Autodesk Fusion 360 part; units mm, degrees
note: some values were not read from the file. Set by a fixed rule: which sketch regions a step uses.
(part 17 of 20)
  spline S37 degree 5 poles (12.6699, 9.771) (12.6679, 9.7705) (12.6637, 9.7696) (12.6575, 9.7682) (12.6492, 9.7663) (12.6389, 9.7639) (12.6286, 9.7615) (12.6184, 9.7591) (12.6081, 9.7566) (12.5979, 9.7542) (12.5878, 9.7518) (12.5776, 9.7493) (12.5675, 9.7469) (12.5574, 9.7444) (12.5474, 9.7419) (12.5374, 9.7394) (12.5274, 9.7369) (12.5174, 9.7344) (12.5075, 9.7319) (12.4976, 9.7293) (12.4877, 9.7268) (12.4779, 9.7243) (12.4681, 9.7217) (12.4583, 9.7191) (12.4486, 9.7166) (12.4389, 9.714) (12.4292, 9.7114) (12.4195, 9.7088) (12.4099, 9.7062) (12.4003, 9.7036) (12.3908, 9.7009) (12.3812, 9.6983) (12.3717, 9.6957) (12.3623, 9.693) (12.3528, 9.6904) (12.3434, 9.6877) (12.3341, 9.685) (12.3247, 9.6823) (12.3154, 9.6797) (12.3062, 9.677) (12.2969, 9.6743) (12.2877, 9.6716) (12.2785, 9.6688) (12.2694, 9.6661) (12.2603, 9.6634) (12.2512, 9.6607) (12.2421, 9.6579) (12.2331, 9.6552) (12.2241, 9.6524) (12.2152, 9.6496) (12.2063, 9.6469) (12.1974, 9.6441) (12.1885, 9.6413) (12.1797, 9.6385) (12.1709, 9.6357) (12.1622, 9.6329) (12.1535, 9.6301) (12.1448, 9.6273) (12.1361, 9.6245) (12.1275, 9.6217) (12.1189, 9.6189) (12.1104, 9.616) (12.1018, 9.6132) (12.0934, 9.6104) (12.0849, 9.6075) (12.0765, 9.6047) (12.0681, 9.6018) (12.0598, 9.599) (12.0515, 9.5961) (12.0432, 9.5933) (12.035, 9.5904) (12.0267, 9.5875) (12.0186, 9.5846) (12.0104, 9.5818) (12.0023, 9.5789) (11.9943, 9.576) (11.9862, 9.5731) (11.9782, 9.5702) (11.9703, 9.5673) (11.9624, 9.5644) (11.9545, 9.5615) (11.9466, 9.5586) (11.9388, 9.5557) (11.931, 9.5528) (11.9233, 9.5499) (11.9156, 9.547) (11.9079, 9.5441) (11.9002, 9.5412) (11.8926, 9.5383) (11.8851, 9.5354) (11.8776, 9.5325) (11.8701, 9.5295) (11.8626, 9.5266) (11.8552, 9.5237) (11.8478, 9.5208) (11.8405, 9.5179) (11.8332, 9.515) (11.8259, 9.512) (11.8187, 9.5091) (11.8115, 9.5062) (11.8043, 9.5033) (11.7972, 9.5004) (11.7901, 9.4975) (11.7831, 9.4945) (11.7761, 9.4916) (11.7691, 9.4887) (11.7622, 9.4858) (11.7553, 9.4829) (11.7484, 9.48) (11.7416, 9.4771) (11.7348, 9.4742) (11.7281, 9.4713) (11.7214, 9.4684) (11.7148, 9.4655) (11.7081, 9.4626) (11.7016, 9.4597) (11.695, 9.4568) (11.6885, 9.4539) (11.6821, 9.451) (11.6756, 9.4482) (11.6693, 9.4453) (11.6629, 9.4424) (11.6566, 9.4396) (11.6504, 9.4367) (11.6441, 9.4338) (11.638, 9.431) (11.6318, 9.4281) (11.6257, 9.4253) (11.6197, 9.4225) (11.6137, 9.4196) (11.6077, 9.4168) (11.6017, 9.414) (11.5959, 9.4112) (11.59, 9.4084) (11.5842, 9.4056) (11.5784, 9.4028) (11.5727, 9.4) (11.567, 9.3972) (11.5614, 9.3944) (11.5558, 9.3917) (11.5502, 9.3889) (11.5447, 9.3862) (11.5392, 9.3834) (11.5338, 9.3807) (11.5284, 9.378) (11.5231, 9.3753) (11.5178, 9.3725) (11.5125, 9.3699) (11.5073, 9.3672) (11.5021, 9.3645) (11.497, 9.3618) (11.4919, 9.3592) (11.4869, 9.3565) (11.4819, 9.3539) (11.4769, 9.3513) (11.472, 9.3487) (11.4672, 9.3461) (11.4623, 9.3435) (11.4576, 9.3409) (11.4528, 9.3383) (11.4482, 9.3358) (11.4435, 9.3332) (11.4389, 9.3307) (11.4344, 9.3282) (11.4299, 9.3257) (11.4254, 9.3232) (11.421, 9.3207) (11.4167, 9.3183) (11.4123, 9.3158) (11.4081, 9.3134) (11.4038, 9.311) (11.3997, 9.3086) (11.3955, 9.3062) (11.3915, 9.3039) (11.3874, 9.3015) (11.3834, 9.2992) (11.3795, 9.2969) (11.3756, 9.2946) (11.3718, 9.2923) (11.368, 9.2901) (11.3642, 9.2878) (11.3605, 9.2856) (11.3569, 9.2834) (11.3533, 9.2812) (11.3497, 9.2791) (11.3462, 9.2769) (11.3428, 9.2748) (11.3394, 9.2727) (11.336, 9.2706) (11.3327, 9.2685) (11.3295, 9.2665) (11.3263, 9.2645) (11.3231, 9.2625) (11.32, 9.2605) (11.317, 9.2586) (11.314, 9.2567) (11.311, 9.2548) (11.3081, 9.2529) (11.3053, 9.2511) (11.3025, 9.2492) (11.2998, 9.2474) (11.2971, 9.2457) (11.2944, 9.2439) (11.2919, 9.2422) (11.2893, 9.2405) (11.2869, 9.2389) (11.2844, 9.2372) (11.2821, 9.2356) (11.2798, 9.2341) (11.2775, 9.2325) (11.2753, 9.231) (11.2732, 9.2295) (11.2711, 9.2281) (11.269, 9.2266) (11.2671, 9.2253) (11.2651, 9.2239) (11.2633, 9.2226) (11.2615, 9.2213) (11.2597, 9.22) (11.258, 9.2188) (11.2564, 9.2177) (11.2548, 9.2165) (11.2533, 9.2154) (11.2518, 9.2143) (11.2504, 9.2133) (11.2491, 9.2123) (11.2478, 9.2113) (11.2465, 9.2104) (11.2454, 9.2096) (11.2443, 9.2087) (11.2432, 9.2079) (11.2422, 9.2072) (11.2413, 9.2065) (11.2404, 9.2058) (11.2396, 9.2052) (11.2389, 9.2046) (11.2382, 9.2041) (11.2376, 9.2036) (11.2371, 9.2032) (11.2366, 9.2028) (11.2362, 9.2025) (11.2359, 9.2022) (11.2357, 9.2021) (11.2356, 9.202) (11.2355, 9.202) knots -1 -1 -1 -1 -1 -1 -0.99583333 -0.99166667 -0.9875 -0.98333333 -0.97916667 -0.975 -0.97083333 -0.96666667 -0.9625 -0.95833333 -0.95416667 -0.95 -0.94583333 -0.94166667 -0.9375 -0.93333333 -0.92916667 -0.925 -0.92083333 -0.91666667 -0.9125 -0.90833333 -0.90416667 -0.9 -0.89583333 -0.89166667 -0.8875 -0.88333333 -0.87916667 -0.875 -0.87083333 -0.86666667 -0.8625 -0.85833333 -0.85416667 -0.85 -0.84583333 -0.84166667 -0.8375 -0.83333333 -0.82916667 -0.825 -0.82083333 -0.81666667 -0.8125 -0.80833333 -0.80416667 -0.8 -0.79583333 -0.79166667 -0.7875 -0.78333333 -0.77916667 -0.775 -0.77083333 -0.76666667 -0.7625 -0.75833333 -0.75416667 -0.75 -0.74583333 -0.74166667 -0.7375 -0.73333333 -0.72916667 -0.725 -0.72083333 -0.71666667 -0.7125 -0.70833333 -0.70416667 -0.7 -0.69583333 -0.69166667 -0.6875 -0.68333333 -0.67916667 -0.675 -0.67083333 -0.66666667 -0.6625 -0.65833333 -0.65416667 -0.65 -0.64583333 -0.64166667 -0.6375 -0.63333333 -0.62916667 -0.625 -0.62083333 -0.61666667 -0.6125 -0.60833333 -0.60416667 -0.6 -0.59583333 -0.59166667 -0.5875 -0.58333333 -0.57916667 -0.575 -0.57083333 -0.56666667 -0.5625 -0.55833333 -0.55416667 -0.55 -0.54583333 -0.54166667 -0.5375 -0.53333333 -0.52916667 -0.525 -0.52083333 -0.51666667 -0.5125 -0.50833333 -0.50416667 -0.5 -0.49583333 -0.49166667 -0.4875 -0.48333333 -0.47916667 -0.475 -0.47083333 -0.46666667 -0.4625 -0.45833333 -0.45416667 -0.45 -0.44583333 -0.44166667 -0.4375 -0.43333333 -0.42916667 -0.425 -0.42083333 -0.41666667 -0.4125 -0.40833333 -0.40416667 -0.4 -0.39583333 -0.39166667 -0.3875 -0.38333333 -0.37916667 -0.375 -0.37083333 -0.36666667 -0.3625 -0.35833333 -0.35416667 -0.35 -0.34583333 -0.34166667 -0.3375 -0.33333333 -0.32916667 -0.325 -0.32083333 -0.31666667 -0.3125 -0.30833333 -0.30416667 -0.3 -0.29583333 -0.29166667 -0.2875 -0.28333333 -0.27916667 -0.275 -0.27083333 -0.26666667 -0.2625 -0.25833333 -0.25416667 -0.25 -0.24583333 -0.24166667 -0.2375 -0.23333333 -0.22916667 -0.225 -0.22083333 -0.21666667 -0.2125 -0.20833333 -0.20416667 -0.2 -0.19583333 -0.19166667 -0.1875 -0.18333333 -0.17916667 -0.175 -0.17083333 -0.16666667 -0.1625 -0.15833333 -0.15416667 -0.15 -0.14583333 -0.14166667 -0.1375 -0.13333333 -0.12916667 -0.125 -0.12083333 -0.11666667 -0.1125 -0.10833333 -0.10416667 -0.1 -0.09583333 -0.09166667 -0.0875 -0.08333333 -0.07916667 -0.075 -0.07083333 -0.06666667 -0.0625 -0.05833333 -0.05416667 -0.05 -0.04583333 -0.04166667 -0.0375 -0.03333333 -0.02916667 -0.025 -0.02083333 -0.01666667 -0.0125 -0.00833333 -0.00416667 0 0 0 0 0 0
  line L74 (11.2355, 9.202) -> (11.235, 9.2016)
  line L75 (11.235, 9.2016) -> (10.6376, 8.7123)
  arc A46 (10.6376, 8.7123) -> (9.7765, 9.6687) centre (0, 0) ccw
  line L76 (9.7765, 9.6687) -> (10.3255, 10.2117)
  line L77 (10.3255, 10.2117) -> (10.326, 10.2121)
  spline S38 degree 5 poles (10.326, 10.2121) (10.326, 10.2122) (10.3261, 10.2123) (10.3263, 10.2124) (10.3266, 10.2127) (10.3269, 10.2131) (10.3274, 10.2135) (10.3279, 10.214) (10.3284, 10.2146) (10.329, 10.2152) (10.3296, 10.2159) (10.3303, 10.2166) (10.3311, 10.2174) (10.3319, 10.2182) (10.3327, 10.2191) (10.3336, 10.2201) (10.3346, 10.2211) (10.3356, 10.2222) (10.3366, 10.2233) (10.3377, 10.2245) (10.3388, 10.2257) (10.34, 10.227) (10.3412, 10.2284) (10.3425, 10.2298) (10.3438, 10.2312) (10.3451, 10.2327) (10.3465, 10.2343) (10.3479, 10.2359) (10.3494, 10.2376) (10.3509, 10.2393) (10.3525, 10.241) (10.354, 10.2429) (10.3557, 10.2447) (10.3573, 10.2467) (10.359, 10.2486) (10.3608, 10.2507) (10.3625, 10.2528) (10.3643, 10.2549) (10.3662, 10.2571) (10.368, 10.2593) (10.37, 10.2616) (10.3719, 10.2639) (10.3739, 10.2663) (10.3759, 10.2688) (10.3779, 10.2712) (10.38, 10.2738) (10.3821, 10.2764) (10.3842, 10.279) (10.3864, 10.2817) (10.3886, 10.2844) (10.3908, 10.2872) (10.3931, 10.29) (10.3954, 10.2929) (10.3977, 10.2958) (10.4, 10.2988) (10.4024, 10.3018) (10.4048, 10.3049) (10.4072, 10.308) (10.4096, 10.3112) (10.4121, 10.3144) (10.4146, 10.3176) (10.4171, 10.3209) (10.4197, 10.3243) (10.4222, 10.3277) (10.4248, 10.3311) (10.4274, 10.3346) (10.4301, 10.3382) (10.4328, 10.3417) (10.4354, 10.3454) (10.4382, 10.349) (10.4409, 10.3528) (10.4436, 10.3565) (10.4464, 10.3603) (10.4492, 10.3642) (10.452, 10.3681) (10.4549, 10.3721) (10.4577, 10.376) (10.4606, 10.3801) (10.4635, 10.3842) (10.4664, 10.3883) (10.4694, 10.3925) (10.4723, 10.3967) (10.4753, 10.4009) (10.4783, 10.4052) (10.4813, 10.4096) (10.4843, 10.414) (10.4874, 10.4184) (10.4904, 10.4229) (10.4935, 10.4274) (10.4966, 10.432) (10.4997, 10.4366) (10.5028, 10.4412) (10.506, 10.4459) (10.5091, 10.4507) (10.5123, 10.4554) (10.5155, 10.4603) (10.5187, 10.4651) (10.5219, 10.47) (10.5251, 10.475) (10.5284, 10.48) (10.5316, 10.485) (10.5349, 10.4901) (10.5382, 10.4952) (10.5415, 10.5003) (10.5448, 10.5055) (10.5481, 10.5108) (10.5515, 10.516) (10.5548, 10.5214) (10.5582, 10.5267) (10.5615, 10.5321) (10.5649, 10.5376) (10.5683, 10.5431) (10.5717, 10.5486) (10.5751, 10.5542) (10.5785, 10.5598) (10.582, 10.5654) (10.5854, 10.5711) (10.5889, 10.5768) (10.5923, 10.5826) (10.5958, 10.5884) (10.5993, 10.5943) (10.6028, 10.6001) (10.6063, 10.6061) (10.6098, 10.612) (10.6133, 10.618) (10.6168, 10.6241) (10.6204, 10.6302) (10.6239, 10.6363) (10.6275, 10.6425) (10.631, 10.6487) (10.6346, 10.6549) (10.6381, 10.6612) (10.6417, 10.6675) (10.6453, 10.6738) (10.6489, 10.6802) (10.6525, 10.6867) (10.6561, 10.6931) (10.6597, 10.6997) (10.6633, 10.7062) (10.6669, 10.7128) (10.6706, 10.7194) (10.6742, 10.7261) (10.6778, 10.7328) (10.6815, 10.7395) (10.6851, 10.7463) (10.6888, 10.7531) (10.6924, 10.7599) (10.6961, 10.7668) (10.6997, 10.7738) (10.7034, 10.7807) (10.7071, 10.7877) (10.7107, 10.7947) (10.7144, 10.8018) (10.7181, 10.8089) (10.7218, 10.8161) (10.7255, 10.8233) (10.7292, 10.8305) (10.7328, 10.8377) (10.7365, 10.845) (10.7402, 10.8523) (10.7439, 10.8597) (10.7476, 10.8671) (10.7513, 10.8745) (10.755, 10.882) (10.7587, 10.8895) (10.7625, 10.8971) (10.7662, 10.9046) (10.7699, 10.9123) (10.7736, 10.9199) (10.7773, 10.9276) (10.781, 10.9353) (10.7847, 10.9431) (10.7884, 10.9509) (10.7921, 10.9587) (10.7958, 10.9666) (10.7996, 10.9745) (10.8033, 10.9824) (10.807, 10.9903) (10.8107, 10.9984) (10.8144, 11.0064) (10.8181, 11.0145) (10.8218, 11.0226) (10.8255, 11.0307) (10.8292, 11.0389) (10.833, 11.0471) (10.8367, 11.0553) (10.8404, 11.0636) (10.8441, 11.0719) (10.8478, 11.0803) (10.8515, 11.0886) (10.8552, 11.097) (10.8589, 11.1055) (10.8625, 11.114) (10.8662, 11.1225) (10.8699, 11.131) (10.8736, 11.1396) (10.8773, 11.1482) (10.881, 11.1569) (10.8847, 11.1655) (10.8883, 11.1743) (10.892, 11.183) (10.8957, 11.1918) (10.8993, 11.2006) (10.903, 11.2094) (10.9066, 11.2183) (10.9103, 11.2272) (10.9139, 11.2362) (10.9176, 11.2451) (10.9212, 11.2541) (10.9249, 11.2632) (10.9285, 11.2723) (10.9321, 11.2814) (10.9358, 11.2905) (10.9394, 11.2997) (10.943, 11.3089) (10.9466, 11.3181) (10.9502, 11.3274) (10.9538, 11.3367) (10.9574, 11.346) (10.961, 11.3553) (10.9646, 11.3647) (10.9682, 11.3742) (10.9717, 11.3836) (10.9753, 11.3931) (10.9789, 11.4026) (10.9824, 11.4122) (10.986, 11.4217) (10.9895, 11.4313) (10.993, 11.441) (10.9966, 11.4507) (11.0001, 11.4604) (11.0036, 11.4701) (11.0071, 11.4799) (11.0106, 11.4897) (11.0141, 11.4995) (11.0176, 11.5093) (11.0211, 11.5192) (11.0246, 11.5291) (11.028, 11.5391) (11.0315, 11.5491) (11.035, 11.5591) (11.0377, 11.5671) (11.0398, 11.5731) (11.0412, 11.5772) (11.0419, 11.5792) knots 0 0 0 0 0 0 0.00416667 0.00833333 0.0125 0.01666667 0.02083333 0.025 0.02916667 0.03333333 0.0375 0.04166667 0.04583333 0.05 0.05416667 0.05833333 0.0625 0.06666667 0.07083333 0.075 0.07916667 0.08333333 0.0875 0.09166667 0.09583333 0.1 0.10416667 0.10833333 0.1125 0.11666667 0.12083333 0.125 0.12916667 0.13333333 0.1375 0.14166667 0.14583333 0.15 0.15416667 0.15833333 0.1625 0.16666667 0.17083333 0.175 0.17916667 0.18333333 0.1875 0.19166667 0.19583333 0.2 0.20416667 0.20833333 0.2125 0.21666667 0.22083333 0.225 0.22916667 0.23333333 0.2375 0.24166667 0.24583333 0.25 0.25416667 0.25833333 0.2625 0.26666667 0.27083333 0.275 0.27916667 0.28333333 0.2875 0.29166667 0.29583333 0.3 0.30416667 0.30833333 0.3125 0.31666667 0.32083333 0.325 0.32916667 0.33333333 0.3375 0.34166667 0.34583333 0.35 0.35416667 0.35833333 0.3625 0.36666667 0.37083333 0.375 0.37916667 0.38333333 0.3875 0.39166667 0.39583333 0.4 0.40416667 0.40833333 0.4125 0.41666667 0.42083333 0.425 0.42916667 0.43333333 0.4375 0.44166667 0.44583333 0.45 0.45416667 0.45833333 0.4625 0.46666667 0.47083333 0.475 0.47916667 0.48333333 0.4875 0.49166667 0.49583333 0.5 0.50416667 0.50833333 0.5125 0.51666667 0.52083333 0.525 0.52916667 0.53333333 0.5375 0.54166667 0.54583333 0.55 0.55416667 0.55833333 0.5625 0.56666667 0.57083333 0.575 0.57916667 0.58333333 0.5875 0.59166667 0.59583333 0.6 0.60416667 0.60833333 0.6125 0.61666667 0.62083333 0.625 0.62916667 0.63333333 0.6375 0.64166667 0.64583333 0.65 0.65416667 0.65833333 0.6625 0.66666667 0.67083333 0.675 0.67916667 0.68333333 0.6875 0.69166667 0.69583333 0.7 0.70416667 0.70833333 0.7125 0.71666667 0.72083333 0.725 0.72916667 0.73333333 0.7375 0.74166667 0.74583333 0.75 0.75416667 0.75833333 0.7625 0.76666667 0.77083333 0.775 0.77916667 0.78333333 0.7875 0.79166667 0.79583333 0.8 0.80416667 0.80833333 0.8125 0.81666667 0.82083333 0.825 0.82916667 0.83333333 0.8375 0.84166667 0.84583333 0.85 0.85416667 0.85833333 0.8625 0.86666667 0.87083333 0.875 0.87916667 0.88333333 0.8875 0.89166667 0.89583333 0.9 0.90416667 0.90833333 0.9125 0.91666667 0.92083333 0.925 0.92916667 0.93333333 0.9375 0.94166667 0.94583333 0.95 0.95416667 0.95833333 0.9625 0.96666667 0.97083333 0.975 0.97916667 0.98333333 0.9875 0.99166667 0.99583333 1 1 1 1 1 1
  arc A47 (11.0419, 11.5792) -> (10.3616, 12.1917) centre (0, 0) ccw
  spline S39 degree 5 poles (10.3616, 12.1917) (10.3596, 12.1908) (10.3558, 12.189) (10.35, 12.1863) (10.3423, 12.1828) (10.3327, 12.1783) (10.3231, 12.1738) (10.3136, 12.1693) (10.3041, 12.1648) (10.2946, 12.1603) (10.2852, 12.1558) (10.2758, 12.1513) (10.2664, 12.1468) (10.2571, 12.1423) (10.2478, 12.1378) (10.2385, 12.1332) (10.2292, 12.1287) (10.22, 12.1242) (10.2108, 12.1197) (10.2017, 12.1151) (10.1925, 12.1106) (10.1834, 12.1061) (10.1744, 12.1015) (10.1654, 12.097) (10.1564, 12.0924) (10.1474, 12.0879) (10.1385, 12.0834) (10.1296, 12.0788) (10.1207, 12.0743) (10.1119, 12.0697) (10.1031, 12.0651) (10.0943, 12.0606) (10.0855, 12.056) (10.0768, 12.0515) (10.0682, 12.0469) (10.0595, 12.0423) (10.0509, 12.0378) (10.0423, 12.0332) (10.0338, 12.0287) (10.0253, 12.0241) (10.0168, 12.0195) (10.0084, 12.015) (9.9999, 12.0104) (9.9916, 12.0058) (9.9832, 12.0013) (9.9749, 11.9967) (9.9666, 11.9921) (9.9584, 11.9876) (9.9502, 11.983) (9.942, 11.9785) (9.9338, 11.9739) (9.9257, 11.9693) (9.9176, 11.9648) (9.9096, 11.9602) (9.9016, 11.9557) (9.8936, 11.9511) (9.8857, 11.9465) (9.8777, 11.942) (9.8699, 11.9374) (9.862, 11.9329) (9.8542, 11.9283) (9.8464, 11.9238) (9.8387, 11.9193) (9.831, 11.9147) (9.8233, 11.9102) (9.8157, 11.9056) (9.8081, 11.9011) (9.8005, 11.8966) (9.793, 11.8921) (9.7855, 11.8875) (9.778, 11.883) (9.7706, 11.8785) (9.7632, 11.874) (9.7558, 11.8695) (9.7485, 11.865) (9.7412, 11.8605) (9.7339, 11.856) (9.7267, 11.8515) (9.7195, 11.847) (9.7124, 11.8425) (9.7053, 11.8381) (9.6982, 11.8336) (9.6912, 11.8291) (9.6841, 11.8247) (9.6772, 11.8202) (9.6702, 11.8158) (9.6633, 11.8113) (9.6565, 11.8069) (9.6496, 11.8025) (9.6428, 11.798) (9.6361, 11.7936) (9.6294, 11.7892) (9.6227, 11.7848) (9.616, 11.7804) (9.6094, 11.776) (9.6028, 11.7717) (9.5963, 11.7673) (9.5898, 11.7629) (9.5833, 11.7586) (9.5769, 11.7542) (9.5705, 11.7499) (9.5642, 11.7455) (9.5578, 11.7412) (9.5516, 11.7369) (9.5453, 11.7326) (9.5391, 11.7283) (9.5329, 11.724) (9.5268, 11.7197) (9.5207, 11.7155) (9.5146, 11.7112) (9.5086, 11.707) (9.5026, 11.7027) (9.4967, 11.6985) (9.4908, 11.6943) (9.4849, 11.6901) (9.4791, 11.6859) (9.4733, 11.6817) (9.4675, 11.6775) (9.4618, 11.6733) (9.4561, 11.6692) (9.4505, 11.6651) (9.4449, 11.6609) (9.4393, 11.6568) (9.4338, 11.6527) (9.4283, 11.6486) (9.4228, 11.6446) (9.4174, 11.6405) (9.412, 11.6365) (9.4067, 11.6324) (9.4014, 11.6284) (9.3962, 11.6244) (9.3909, 11.6204) (9.3858, 11.6164) (9.3806, 11.6125) (9.3755, 11.6085) (9.3705, 11.6046) (9.3654, 11.6007) (9.3605, 11.5968) (9.3555, 11.5929) (9.3506, 11.589) (9.3457, 11.5852) (9.3409, 11.5813) (9.3361, 11.5775) (9.3314, 11.5737) (9.3267, 11.5699) (9.322, 11.5662) (9.3174, 11.5624) (9.3128, 11.5587) (9.3083, 11.555) (9.3038, 11.5513) (9.2993, 11.5476) (9.2949, 11.544) (9.2905, 11.5403) (9.2862, 11.5367) (9.2819, 11.5331) (9.2776, 11.5295) (9.2734, 11.526) (9.2692, 11.5224) (9.2651, 11.5189) (9.261, 11.5154) (9.257, 11.512) (9.253, 11.5085) (9.249, 11.5051) (9.2451, 11.5017) (9.2412, 11.4983) (9.2373, 11.495) (9.2335, 11.4916) (9.2298, 11.4883) (9.2261, 11.485) (9.2224, 11.4818) (9.2188, 11.4785) (9.2152, 11.4753) (9.2116, 11.4721) (9.2081, 11.469) (9.2047, 11.4658) (9.2013, 11.4627) (9.1979, 11.4597) (9.1946, 11.4566) (9.1913, 11.4536) (9.188, 11.4506) (9.1848, 11.4476) (9.1817, 11.4447) (9.1786, 11.4418) (9.1755, 11.4389) (9.1725, 11.436) (9.1695, 11.4332) (9.1666, 11.4304) (9.1637, 11.4276) (9.1608, 11.4249) (9.158, 11.4222) (9.1553, 11.4195) (9.1526, 11.4169) (9.1499, 11.4143) (9.1473, 11.4117) (9.1447, 11.4092) (9.1422, 11.4067) (9.1397, 11.4042) (9.1372, 11.4018) (9.1348, 11.3994) (9.1325, 11.397) (9.1302, 11.3947) (9.1279, 11.3924) (9.1257, 11.3902) (9.1235, 11.388) (9.1214, 11.3858) (9.1194, 11.3836) (9.1173, 11.3815) (9.1153, 11.3795) (9.1134, 11.3775) (9.1115, 11.3755) (9.1097, 11.3735) (9.1079, 11.3717) (9.1062, 11.3698) (9.1045, 11.368) (9.1028, 11.3662) (9.1012, 11.3645) (9.0997, 11.3628) (9.0982, 11.3612) (9.0967, 11.3596) (9.0953, 11.3581) (9.0939, 11.3566) (9.0926, 11.3551) (9.0914, 11.3537) (9.0902, 11.3524) (9.089, 11.3511) (9.0879, 11.3498) (9.0868, 11.3486) (9.0858, 11.3475) (9.0849, 11.3464) (9.084, 11.3453) (9.0831, 11.3443) (9.0823, 11.3434) (9.0815, 11.3425) (9.0808, 11.3417) (9.0802, 11.3409) (9.0796, 11.3402) (9.079, 11.3395) (9.0785, 11.3389) (9.0781, 11.3384) (9.0777, 11.3379) (9.0773, 11.3375) (9.0771, 11.3372) (9.0769, 11.337) (9.0769, 11.3369) (9.0768, 11.3369) knots -1 -1 -1 -1 -1 -1 -0.99583333 -0.99166667 -0.9875 -0.98333333 -0.97916667 -0.975 -0.97083333 -0.96666667 -0.9625 -0.95833333 -0.95416667 -0.95 -0.94583333 -0.94166667 -0.9375 -0.93333333 -0.92916667 -0.925 -0.92083333 -0.91666667 -0.9125 -0.90833333 -0.90416667 -0.9 -0.89583333 -0.89166667 -0.8875 -0.88333333 -0.87916667 -0.875 -0.87083333 -0.86666667 -0.8625 -0.85833333 -0.85416667 -0.85 -0.84583333 -0.84166667 -0.8375 -0.83333333 -0.82916667 -0.825 -0.82083333 -0.81666667 -0.8125 -0.80833333 -0.80416667 -0.8 -0.79583333 -0.79166667 -0.7875 -0.78333333 -0.77916667 -0.775 -0.77083333 -0.76666667 -0.7625 -0.75833333 -0.75416667 -0.75 -0.74583333 -0.74166667 -0.7375 -0.73333333 -0.72916667 -0.725 -0.72083333 -0.71666667 -0.7125 -0.70833333 -0.70416667 -0.7 -0.69583333 -0.69166667 -0.6875 -0.68333333 -0.67916667 -0.675 -0.67083333 -0.66666667 -0.6625 -0.65833333 -0.65416667 -0.65 -0.64583333 -0.64166667 -0.6375 -0.63333333 -0.62916667 -0.625 -0.62083333 -0.61666667 -0.6125 -0.60833333 -0.60416667 -0.6 -0.59583333 -0.59166667 -0.5875 -0.58333333 -0.57916667 -0.575 -0.57083333 -0.56666667 -0.5625 -0.55833333 -0.55416667 -0.55 -0.54583333 -0.54166667 -0.5375 -0.53333333 -0.52916667 -0.525 -0.52083333 -0.51666667 -0.5125 -0.50833333 -0.50416667 -0.5 -0.49583333 -0.49166667 -0.4875 -0.48333333 -0.47916667 -0.475 -0.47083333 -0.46666667 -0.4625 -0.45833333 -0.45416667 -0.45 -0.44583333 -0.44166667 -0.4375 -0.43333333 -0.42916667 -0.425 -0.42083333 -0.41666667 -0.4125 -0.40833333 -0.40416667 -0.4 -0.39583333 -0.39166667 -0.3875 -0.38333333 -0.37916667 -0.375 -0.37083333 -0.36666667 -0.3625 -0.35833333 -0.35416667 -0.35 -0.34583333 -0.34166667 -0.3375 -0.33333333 -0.32916667 -0.325 -0.32083333 -0.31666667 -0.3125 -0.30833333 -0.30416667 -0.3 -0.29583333 -0.29166667 -0.2875 -0.28333333 -0.27916667 -0.275 -0.27083333 -0.26666667 -0.2625 -0.25833333 -0.25416667 -0.25 -0.24583333 -0.24166667 -0.2375 -0.23333333 -0.22916667 -0.225 -0.22083333 -0.21666667 -0.2125 -0.20833333 -0.20416667 -0.2 -0.19583333 -0.19166667 -0.1875 -0.18333333 -0.17916667 -0.175 -0.17083333 -0.16666667 -0.1625 -0.15833333 -0.15416667 -0.15 -0.14583333 -0.14166667 -0.1375 -0.13333333 -0.12916667 -0.125 -0.12083333 -0.11666667 -0.1125 -0.10833333 -0.10416667 -0.1 -0.09583333 -0.09166667 -0.0875 -0.08333333 -0.07916667 -0.075 -0.07083333 -0.06666667 -0.0625 -0.05833333 -0.05416667 -0.05 -0.04583333 -0.04166667 -0.0375 -0.03333333 -0.02916667 -0.025 -0.02083333 -0.01666667 -0.0125 -0.00833333 -0.00416667 0 0 0 0 0 0
  line L78 (9.0768, 11.3369) -> (9.0764, 11.3364)
  line L79 (9.0764, 11.3364) -> (8.5938, 10.7336)
  arc A48 (8.5938, 10.7336) -> (7.5526, 11.49) centre (0, 0) ccw
  line L80 (7.5526, 11.49) -> (7.9768, 12.1353)
  line L81 (7.9768, 12.1353) -> (7.9771, 12.1359)
  spline S40 degree 5 poles (7.9771, 12.1359) (7.9772, 12.1359) (7.9772, 12.136) (7.9774, 12.1362) (7.9776, 12.1365) (7.9779, 12.137) (7.9782, 12.1375) (7.9786, 12.1381) (7.979, 12.1388) (7.9794, 12.1395) (7.9799, 12.1403) (7.9804, 12.1411) (7.981, 12.1421) (7.9816, 12.1431) (7.9823, 12.1441) (7.9829, 12.1452) (7.9836, 12.1464) (7.9844, 12.1477) (7.9852, 12.149) (7.986, 12.1504) (7.9868, 12.1518) (7.9877, 12.1533) (7.9886, 12.1549) (7.9896, 12.1565) (7.9905, 12.1582) (7.9915, 12.16) (7.9926, 12.1618) (7.9936, 12.1637) (7.9947, 12.1656) (7.9958, 12.1676) (7.997, 12.1696) (7.9982, 12.1718) (7.9994, 12.1739) (8.0006, 12.1762) (8.0018, 12.1785) (8.0031, 12.1808) (8.0044, 12.1832) (8.0057, 12.1857) (8.0071, 12.1882) (8.0084, 12.1908) (8.0098, 12.1934) (8.0113, 12.1961) (8.0127, 12.1988) (8.0142, 12.2016) (8.0156, 12.2045) (8.0171, 12.2074) (8.0187, 12.2104) (8.0202, 12.2134) (8.0218, 12.2164) (8.0233, 12.2196) (8.0249, 12.2228) (8.0265, 12.226) (8.0282, 12.2293) (8.0298, 12.2326) (8.0315, 12.236) (8.0332, 12.2395) (8.0349, 12.243) (8.0366, 12.2465) (8.0383, 12.2501) (8.0401, 12.2538) (8.0419, 12.2575) (8.0436, 12.2612) (8.0454, 12.265) (8.0472, 12.2689) (8.0491, 12.2728) (8.0509, 12.2768) (8.0527, 12.2808) (8.0546, 12.2848) (8.0565, 12.289) (8.0584, 12.2931) (8.0603, 12.2973) (8.0622, 12.3016) (8.0641, 12.3059) (8.066, 12.3102) (8.068, 12.3146) (8.0699, 12.3191) (8.0719, 12.3236) (8.0739, 12.3281) (8.0759, 12.3327) (8.0779, 12.3374) (8.0799, 12.3421) (8.0819, 12.3468) (8.0839, 12.3516) (8.0859, 12.3564) (8.088, 12.3613) (8.09, 12.3662) (8.0921, 12.3712) (8.0941, 12.3762) (8.0962, 12.3813) (8.0983, 12.3864) (8.1004, 12.3915) (8.1025, 12.3967) (8.1046, 12.402) (8.1067, 12.4073) (8.1088, 12.4126) (8.1109, 12.418) (8.113, 12.4234) (8.1151, 12.4289) (8.1173, 12.4344) (8.1194, 12.4399) (8.1215, 12.4455) (8.1237, 12.4512) (8.1258, 12.4568) (8.128, 12.4626) (8.1302, 12.4683) (8.1323, 12.4742) (8.1345, 12.48) (8.1366, 12.4859) (8.1388, 12.4919) (8.141, 12.4979) (8.1432, 12.5039) (8.1453, 12.51) (8.1475, 12.5161) (8.1497, 12.5222) (8.1519, 12.5284) (8.1541, 12.5347) (8.1563, 12.5409) (8.1584, 12.5473) (8.1606, 12.5536) (8.1628, 12.56) (8.165, 12.5665) (8.1672, 12.5729) (8.1694, 12.5795) (8.1716, 12.586) (8.1738, 12.5926) (8.176, 12.5993) (8.1782, 12.606) (8.1803, 12.6127) (8.1825, 12.6195) (8.1847, 12.6263) (8.1869, 12.6331) (8.1891, 12.64) (8.1913, 12.6469) (8.1935, 12.6539) (8.1956, 12.6609) (8.1978, 12.6679) (8.2, 12.675) (8.2022, 12.6821) (8.2044, 12.6893) (8.2065, 12.6965) (8.2087, 12.7037) (8.2109, 12.711) (8.213, 12.7183) (8.2152, 12.7256) (8.2173, 12.733) (8.2195, 12.7404) (8.2216, 12.7479) (8.2238, 12.7554) (8.2259, 12.7629) (8.2281, 12.7705) (8.2302, 12.7781) (8.2323, 12.7857) (8.2345, 12.7934) (8.2366, 12.8011) (8.2387, 12.8089) (8.2408, 12.8167) (8.2429, 12.8245) (8.245, 12.8324) (8.2471, 12.8403) (8.2492, 12.8482) (8.2513, 12.8562) (8.2534, 12.8642) (8.2554, 12.8722) (8.2575, 12.8803) (8.2596, 12.8884) (8.2616, 12.8966) (8.2637, 12.9048) (8.2657, 12.913) (8.2678, 12.9212) (8.2698, 12.9295) (8.2718, 12.9379) (8.2738, 12.9462) (8.2759, 12.9546) (8.2779, 12.963) (8.2799, 12.9715) (8.2818, 12.98) (8.2838, 12.9885) (8.2858, 12.9971) (8.2878, 13.0057) (8.2897, 13.0143) (8.2917, 13.023) (8.2936, 13.0317) (8.2956, 13.0404) (8.2975, 13.0492) (8.2994, 13.058) (8.3013, 13.0668) (8.3032, 13.0757) (8.3051, 13.0846) (8.307, 13.0935) (8.3089, 13.1025) (8.3107, 13.1115) (8.3126, 13.1205) (8.3145, 13.1296) (8.3163, 13.1386) (8.3181, 13.1478) (8.3199, 13.1569) (8.3218, 13.1661) (8.3236, 13.1753) (8.3254, 13.1846) (8.3271, 13.1939) (8.3289, 13.2032) (8.3307, 13.2125) (8.3324, 13.2219) (8.3342, 13.2313) (8.3359, 13.2408) (8.3376, 13.2503) (8.3393, 13.2598) (8.341, 13.2693) (8.3427, 13.2789) (8.3444, 13.2885) (8.3461, 13.2981) (8.3477, 13.3078) (8.3494, 13.3174) (8.351, 13.3272) (8.3526, 13.3369) (8.3542, 13.3467) (8.3558, 13.3565) (8.3574, 13.3663) (8.359, 13.3762) (8.3606, 13.3861) (8.3621, 13.396) (8.3637, 13.406) (8.3652, 13.416) (8.3667, 13.426) (8.3682, 13.4361) (8.3697, 13.4461) (8.3712, 13.4563) (8.3726, 13.4664) (8.3741, 13.4766) (8.3755, 13.4867) (8.377, 13.497) (8.3784, 13.5072) (8.3798, 13.5175) (8.3812, 13.5278) (8.3826, 13.5382) (8.3839, 13.5485) (8.3853, 13.5589) (8.3866, 13.5693) (8.3879, 13.5798) (8.3893, 13.5903) (8.3906, 13.6008) (8.3916, 13.6092) (8.3924, 13.6155) (8.3929, 13.6198) (8.3931, 13.6219) knots 0 0 0 0 0 0 0.00416667 0.00833333 0.0125 0.01666667 0.02083333 0.025 0.02916667 0.03333333 0.0375 0.04166667 0.04583333 0.05 0.05416667 0.05833333 0.0625 0.06666667 0.07083333 0.075 0.07916667 0.08333333 0.0875 0.09166667 0.09583333 0.1 0.10416667 0.10833333 0.1125 0.11666667 0.12083333 0.125 0.12916667 0.13333333 0.1375 0.14166667 0.14583333 0.15 0.15416667 0.15833333 0.1625 0.16666667 0.17083333 0.175 0.17916667 0.18333333 0.1875 0.19166667 0.19583333 0.2 0.20416667 0.20833333 0.2125 0.21666667 0.22083333 0.225 0.22916667 0.23333333 0.2375 0.24166667 0.24583333 0.25 0.25416667 0.25833333 0.2625 0.26666667 0.27083333 0.275 0.27916667 0.28333333 0.2875 0.29166667 0.29583333 0.3 0.30416667 0.30833333 0.3125 0.31666667 0.32083333 0.325 0.32916667 0.33333333 0.3375 0.34166667 0.34583333 0.35 0.35416667 0.35833333 0.3625 0.36666667 0.37083333 0.375 0.37916667 0.38333333 0.3875 0.39166667 0.39583333 0.4 0.40416667 0.40833333 0.4125 0.41666667 0.42083333 0.425 0.42916667 0.43333333 0.4375 0.44166667 0.44583333 0.45 0.45416667 0.45833333 0.4625 0.46666667 0.47083333 0.475 0.47916667 0.48333333 0.4875 0.49166667 0.49583333 0.5 0.50416667 0.50833333 0.5125 0.51666667 0.52083333 0.525 0.52916667 0.53333333 0.5375 0.54166667 0.54583333 0.55 0.55416667 0.55833333 0.5625 0.56666667 0.57083333 0.575 0.57916667 0.58333333 0.5875 0.59166667 0.59583333 0.6 0.60416667 0.60833333 0.6125 0.61666667 0.62083333 0.625 0.62916667 0.63333333 0.6375 0.64166667 0.64583333 0.65 0.65416667 0.65833333 0.6625 0.66666667 0.67083333 0.675 0.67916667 0.68333333 0.6875 0.69166667 0.69583333 0.7 0.70416667 0.70833333 0.7125 0.71666667 0.72083333 0.725 0.72916667 0.73333333 0.7375 0.74166667 0.74583333 0.75 0.75416667 0.75833333 0.7625 0.76666667 0.77083333 0.775 0.77916667 0.78333333 0.7875 0.79166667 0.79583333 0.8 0.80416667 0.80833333 0.8125 0.81666667 0.82083333 0.825 0.82916667 0.83333333 0.8375 0.84166667 0.84583333 0.85 0.85416667 0.85833333 0.8625 0.86666667 0.87083333 0.875 0.87916667 0.88333333 0.8875 0.89166667 0.89583333 0.9 0.90416667 0.90833333 0.9125 0.91666667 0.92083333 0.925 0.92916667 0.93333333 0.9375 0.94166667 0.94583333 0.95 0.95416667 0.95833333 0.9625 0.96666667 0.97083333 0.975 0.97916667 0.98333333 0.9875 0.99166667 0.99583333 1 1 1 1 1 1
  arc A49 (8.3931, 13.6219) -> (7.6003, 14.0796) centre (0, 0) ccw
  spline S41 degree 5 poles (7.6003, 14.0796) (7.5986, 14.0783) (7.5952, 14.0758) (7.5901, 14.0719) (7.5833, 14.0668) (7.5749, 14.0604) (7.5665, 14.0541) (7.5581, 14.0477) (7.5497, 14.0413) (7.5414, 14.035) (7.5331, 14.0286) (7.5248, 14.0222) (7.5166, 14.0159) (7.5084, 14.0095) (7.5002, 14.0032) (7.4921, 13.9968) (7.484, 13.9905) (7.4759, 13.9841) (7.4679, 13.9778) (7.4599, 13.9714) (7.4519, 13.9651) (7.4439, 13.9588) (7.436, 13.9525) (7.4281, 13.9461) (7.4203, 13.9398) (7.4124, 13.9335) (7.4046, 13.9272) (7.3969, 13.9209) (7.3892, 13.9146) (7.3815, 13.9083) (7.3738, 13.902) (7.3662, 13.8958) (7.3586, 13.8895) (7.351, 13.8832) (7.3435, 13.8769) (7.336, 13.8707) (7.3285, 13.8644) (7.321, 13.8582) (7.3136, 13.8519) (7.3063, 13.8457) (7.2989, 13.8395) (7.2916, 13.8333) (7.2843, 13.827) (7.2771, 13.8208) (7.2699, 13.8146) (7.2627, 13.8084) (7.2555, 13.8023) (7.2484, 13.7961) (7.2413, 13.7899) (7.2343, 13.7837) (7.2272, 13.7776) (7.2203, 13.7714) (7.2133, 13.7653) (7.2064, 13.7592) (7.1995, 13.753) (7.1926, 13.7469) (7.1858, 13.7408) (7.179, 13.7347) (7.1723, 13.7286) (7.1655, 13.7226) (7.1588, 13.7165) (7.1522, 13.7104) (7.1455, 13.7044) (7.1389, 13.6983) (7.1324, 13.6923) (7.1259, 13.6863) (7.1194, 13.6803) (7.1129, 13.6743) (7.1065, 13.6683) (7.1001, 13.6623) (7.0937, 13.6563) (7.0874, 13.6504) (7.0811, 13.6444) (7.0748, 13.6385) (7.0686, 13.6325) (7.0624, 13.6266) (7.0562, 13.6207) (7.0501, 13.6148) (7.044, 13.6089) (7.0379, 13.6031) (7.0319, 13.5972) (7.0259, 13.5914) (7.02, 13.5855) (7.014, 13.5797) (7.0081, 13.5739) (7.0023, 13.5681) (6.9965, 13.5624) (6.9907, 13.5566) (6.9849, 13.5508) (6.9792, 13.5451) (6.9735, 13.5394) (6.9678, 13.5337) (6.9622, 13.528) (6.9566, 13.5223) (6.9511, 13.5166) (6.9455, 13.511) (6.94, 13.5053) (6.9346, 13.4997) (6.9292, 13.4941) (6.9238, 13.4885) (6.9184, 13.4829) (6.9131, 13.4774) (6.9078, 13.4718) (6.9026, 13.4663) (6.8974, 13.4608) (6.8922, 13.4553) (6.8871, 13.4498) (6.8819, 13.4444) (6.8769, 13.4389) (6.8718, 13.4335) (6.8668, 13.4281) (6.8618, 13.4227) (6.8569, 13.4173) (6.852, 13.412) (6.8471, 13.4066) (6.8423, 13.4013) (6.8375, 13.396) (6.8327, 13.3907) (6.828, 13.3855) (6.8233, 13.3802) (6.8187, 13.375) (6.814, 13.3698) (6.8094, 13.3646) (6.8049, 13.3595) (6.8004, 13.3543) (6.7959, 13.3492) (6.7914, 13.3441) (6.787, 13.339) (6.7826, 13.334) (6.7783, 13.329) (6.774, 13.3239) (6.7697, 13.319) (6.7655, 13.314) (6.7613, 13.309) (6.7571, 13.3041) (6.753, 13.2992) (6.7489, 13.2944) (6.7448, 13.2895) (6.7408, 13.2847) (6.7368, 13.2799) (6.7328, 13.2751) (6.7289, 13.2703) (6.725, 13.2656) (6.7212, 13.2609) (6.7174, 13.2562) (6.7136, 13.2516) (6.7098, 13.2469) (6.7061, 13.2423) (6.7025, 13.2378) (6.6988, 13.2332) (6.6952, 13.2287) (6.6917, 13.2242) (6.6881, 13.2197) (6.6846, 13.2153) (6.6812, 13.2109) (6.6778, 13.2065) (6.6744, 13.2022) (6.671, 13.1978) (6.6677, 13.1935) (6.6644, 13.1893) (6.6612, 13.185) (6.658, 13.1808) (6.6548, 13.1767) (6.6517, 13.1725) (6.6486, 13.1684) (6.6455, 13.1643) (6.6425, 13.1603) (6.6395, 13.1563) (6.6366, 13.1523) (6.6337, 13.1483) (6.6308, 13.1444) (6.628, 13.1405) (6.6252, 13.1367) (6.6224, 13.1328) (6.6197, 13.1291) (6.617, 13.1253) (6.6143, 13.1216) (6.6117, 13.1179) (6.6091, 13.1143) (6.6065, 13.1107) (6.604, 13.1071) (6.6016, 13.1036) (6.5991, 13.1001) (6.5967, 13.0966) (6.5944, 13.0932) (6.592, 13.0898) (6.5897, 13.0865) (6.5875, 13.0832) (6.5853, 13.0799) (6.5831, 13.0767) (6.581, 13.0735) (6.5788, 13.0703) (6.5768, 13.0672) (6.5747, 13.0642) (6.5728, 13.0612) (6.5708, 13.0582) (6.5689, 13.0553) (6.567, 13.0524) (6.5651, 13.0495) (6.5633, 13.0467) (6.5616, 13.044) (6.5598, 13.0413) (6.5581, 13.0386) (6.5565, 13.036) (6.5549, 13.0334) (6.5533, 13.0309) (6.5517, 13.0284) (6.5502, 13.026) (6.5488, 13.0236) (6.5473, 13.0213) (6.5459, 13.019) (6.5446, 13.0168) (6.5433, 13.0146) (6.542, 13.0125) (6.5407, 13.0104) (6.5395, 13.0084) (6.5384, 13.0064) (6.5372, 13.0045) (6.5361, 13.0027) (6.5351, 13.0009) (6.5341, 12.9991) (6.5331, 12.9974) (6.5321, 12.9958) (6.5312, 12.9942) (6.5304, 12.9927) (6.5295, 12.9913) (6.5288, 12.9899) (6.528, 12.9885) (6.5273, 12.9873) (6.5266, 12.986) (6.526, 12.9849) (6.5254, 12.9838) (6.5248, 12.9828) (6.5243, 12.9818) (6.5238, 12.9809) (6.5234, 12.9801) (6.523, 12.9794) (6.5226, 12.9787) (6.5223, 12.9781) (6.522, 12.9775) (6.5218, 12.977) (6.5216, 12.9767) (6.5215, 12.9765) (6.5214, 12.9764) (6.5214, 12.9763) knots -1 -1 -1 -1 -1 -1 -0.99583333 -0.99166667 -0.9875 -0.98333333 -0.97916667 -0.975 -0.97083333 -0.96666667 -0.9625 -0.95833333 -0.95416667 -0.95 -0.94583333 -0.94166667 -0.9375 -0.93333333 -0.92916667 -0.925 -0.92083333 -0.91666667 -0.9125 -0.90833333 -0.90416667 -0.9 -0.89583333 -0.89166667 -0.8875 -0.88333333 -0.87916667 -0.875 -0.87083333 -0.86666667 -0.8625 -0.85833333 -0.85416667 -0.85 -0.84583333 -0.84166667 -0.8375 -0.83333333 -0.82916667 -0.825 -0.82083333 -0.81666667 -0.8125 -0.80833333 -0.80416667 -0.8 -0.79583333 -0.79166667 -0.7875 -0.78333333 -0.77916667 -0.775 -0.77083333 -0.76666667 -0.7625 -0.75833333 -0.75416667 -0.75 -0.74583333 -0.74166667 -0.7375 -0.73333333 -0.72916667 -0.725 -0.72083333 -0.71666667 -0.7125 -0.70833333 -0.70416667 -0.7 -0.69583333 -0.69166667 -0.6875 -0.68333333 -0.67916667 -0.675 -0.67083333 -0.66666667 -0.6625 -0.65833333 -0.65416667 -0.65 -0.64583333 -0.64166667 -0.6375 -0.63333333 -0.62916667 -0.625 -0.62083333 -0.61666667 -0.6125 -0.60833333 -0.60416667 -0.6 -0.59583333 -0.59166667 -0.5875 -0.58333333 -0.57916667 -0.575 -0.57083333 -0.56666667 -0.5625 -0.55833333 -0.55416667 -0.55 -0.54583333 -0.54166667 -0.5375 -0.53333333 -0.52916667 -0.525 -0.52083333 -0.51666667 -0.5125 -0.50833333 -0.50416667 -0.5 -0.49583333 -0.49166667 -0.4875 -0.48333333 -0.47916667 -0.475 -0.47083333 -0.46666667 -0.4625 -0.45833333 -0.45416667 -0.45 -0.44583333 -0.44166667 -0.4375 -0.43333333 -0.42916667 -0.425 -0.42083333 -0.41666667 -0.4125 -0.40833333 -0.40416667 -0.4 -0.39583333 -0.39166667 -0.3875 -0.38333333 -0.37916667 -0.375 -0.37083333 -0.36666667 -0.3625 -0.35833333 -0.35416667 -0.35 -0.34583333 -0.34166667 -0.3375 -0.33333333 -0.32916667 -0.325 -0.32083333 -0.31666667 -0.3125 -0.30833333 -0.30416667 -0.3 -0.29583333 -0.29166667 -0.2875 -0.28333333 -0.27916667 -0.275 -0.27083333 -0.26666667 -0.2625 -0.25833333 -0.25416667 -0.25 -0.24583333 -0.24166667 -0.2375 -0.23333333 -0.22916667 -0.225 -0.22083333 -0.21666667 -0.2125 -0.20833333 -0.20416667 -0.2 -0.19583333 -0.19166667 -0.1875 -0.18333333 -0.17916667 -0.175 -0.17083333 -0.16666667 -0.1625 -0.15833333 -0.15416667 -0.15 -0.14583333 -0.14166667 -0.1375 -0.13333333 -0.12916667 -0.125 -0.12083333 -0.11666667 -0.1125 -0.10833333 -0.10416667 -0.1 -0.09583333 -0.09166667 -0.0875 -0.08333333 -0.07916667 -0.075 -0.07083333 -0.06666667 -0.0625 -0.05833333 -0.05416667 -0.05 -0.04583333 -0.04166667 -0.0375 -0.03333333 -0.02916667 -0.025 -0.02083333 -0.01666667 -0.0125 -0.00833333 -0.00416667 0 0 0 0 0 0
  line L82 (6.5214, 12.9763) -> (6.5211, 12.9757)
  line L83 (6.5211, 12.9757) -> (6.1743, 12.2858)
  arc A50 (6.1743, 12.2858) -> (4.9987, 12.8092) centre (0, 0) ccw
  line L84 (4.9987, 12.8092) -> (5.2794, 13.5286)
  line L85 (5.2794, 13.5286) -> (5.2796, 13.5292)
  spline S42 degree 5 poles (5.2796, 13.5292) (5.2796, 13.5293) (5.2797, 13.5294) (5.2798, 13.5296) (5.2799, 13.53) (5.2801, 13.5305) (5.2803, 13.531) (5.2805, 13.5317) (5.2808, 13.5324) (5.2811, 13.5332) (5.2814, 13.5341) (5.2818, 13.5351) (5.2821, 13.5361) (5.2825, 13.5372) (5.2829, 13.5383) (5.2833, 13.5396) (5.2838, 13.5409) (5.2843, 13.5423) (5.2848, 13.5437) (5.2853, 13.5452) (5.2858, 13.5468) (5.2863, 13.5485) (5.2869, 13.5502) (5.2875, 13.552) (5.2881, 13.5539) (5.2887, 13.5558) (5.2893, 13.5578) (5.29, 13.5598) (5.2907, 13.5619) (5.2913, 13.5641) (5.292, 13.5664) (5.2927, 13.5687) (5.2935, 13.5711) (5.2942, 13.5735) (5.2949, 13.576) (5.2957, 13.5786) (5.2965, 13.5812) (5.2972, 13.5839) (5.298, 13.5866) (5.2988, 13.5894) (5.2997, 13.5923) (5.3005, 13.5952) (5.3013, 13.5982) (5.3022, 13.6012) (5.303, 13.6043) (5.3039, 13.6075) (5.3047, 13.6107) (5.3056, 13.614) (5.3065, 13.6173) (5.3074, 13.6207) (5.3083, 13.6241) (5.3092, 13.6276) (5.3101, 13.6312) (5.3111, 13.6348) (5.312, 13.6385) (5.3129, 13.6422) (5.3138, 13.646) (5.3148, 13.6498) (5.3157, 13.6537) (5.3167, 13.6576) (5.3176, 13.6616) (5.3186, 13.6657) (5.3196, 13.6698) (5.3205, 13.6739) (5.3215, 13.6781) (5.3225, 13.6824) (5.3235, 13.6867) (5.3244, 13.691) (5.3254, 13.6954) (5.3264, 13.6999) (5.3274, 13.7044) (5.3284, 13.709) (5.3293, 13.7136) (5.3303, 13.7183) (5.3313, 13.723) (5.3323, 13.7277) (5.3333, 13.7325) (5.3343, 13.7374) (5.3353, 13.7423) (5.3363, 13.7473) (5.3372, 13.7523) (5.3382, 13.7573) (5.3392, 13.7624) (5.3402, 13.7676) (5.3412, 13.7728) (5.3422, 13.778) (5.3431, 13.7833) (5.3441, 13.7886) (5.3451, 13.794) (5.3461, 13.7994) (5.347, 13.8049) (5.348, 13.8104) (5.3489, 13.816) (5.3499, 13.8216) (5.3509, 13.8273) (5.3518, 13.833) (5.3528, 13.8387) (5.3537, 13.8445) (5.3546, 13.8503) (5.3556, 13.8562) (5.3565, 13.8621) (5.3574, 13.8681) (5.3583, 13.8741) (5.3593, 13.8801) (5.3602, 13.8862) (5.3611, 13.8924) (5.362, 13.8986) (5.3629, 13.9048) (5.3638, 13.911) (5.3646, 13.9173) (5.3655, 13.9237) (5.3664, 13.9301) (5.3672, 13.9365) (5.3681, 13.943) (5.3689, 13.9495) (5.3698, 13.9561) (5.3706, 13.9627) (5.3714, 13.9693) (5.3723, 13.976) (5.3731, 13.9827) (5.3739, 13.9895) (5.3747, 13.9963) (5.3755, 14.0031) (5.3762, 14.01) (5.377, 14.0169) (5.3778, 14.0238) (5.3785, 14.0308) (5.3793, 14.0379) (5.38, 14.0449) (5.3807, 14.0521) (5.3814, 14.0592) (5.3821, 14.0664) (5.3828, 14.0736) (5.3835, 14.0809) (5.3842, 14.0882) (5.3849, 14.0955) (5.3855, 14.1029) (5.3862, 14.1103) (5.3868, 14.1178) (5.3874, 14.1253) (5.3881, 14.1328) (5.3887, 14.1403) (5.3893, 14.1479) (5.3899, 14.1556) (5.3904, 14.1632) (5.391, 14.171) (5.3915, 14.1787) (5.3921, 14.1865) (5.3926, 14.1943) (5.3931, 14.2021) (5.3936, 14.21) (5.3941, 14.2179) (5.3946, 14.2259) (5.3951, 14.2339) (5.3955, 14.2419) (5.396, 14.25) (5.3964, 14.2581) (5.3968, 14.2662) (5.3973, 14.2744) (5.3976, 14.2826) (5.398, 14.2908) (5.3984, 14.2991) (5.3988, 14.3074) (5.3991, 14.3157) (5.3994, 14.3241) (5.3998, 14.3325) (5.4001, 14.3409) (5.4003, 14.3493) (5.4006, 14.3578) (5.4009, 14.3664) (5.4011, 14.3749) (5.4014, 14.3835) (5.4016, 14.3922) (5.4018, 14.4008) (5.402, 14.4095) (5.4022, 14.4182) (5.4023, 14.427) (5.4025, 14.4358) (5.4026, 14.4446) (5.4028, 14.4535) (5.4029, 14.4623) (5.403, 14.4712) (5.403, 14.4802) (5.4031, 14.4892) (5.4031, 14.4982) (5.4032, 14.5072) (5.4032, 14.5163) (5.4032, 14.5254) (5.4032, 14.5345) (5.4032, 14.5437) (5.4031, 14.5528) (5.4031, 14.5621) (5.403, 14.5713) (5.4029, 14.5806) (5.4028, 14.5899) (5.4027, 14.5992) (5.4025, 14.6086) (5.4024, 14.618) (5.4022, 14.6274) (5.402, 14.6369) (5.4018, 14.6464) (5.4016, 14.6559) (5.4013, 14.6654) (5.4011, 14.675) (5.4008, 14.6846) (5.4005, 14.6942) (5.4002, 14.7038) (5.3999, 14.7135) (5.3996, 14.7232) (5.3992, 14.733) (5.3988, 14.7427) (5.3985, 14.7525) (5.3981, 14.7624) (5.3976, 14.7722) (5.3972, 14.7821) (5.3967, 14.792) (5.3963, 14.8019) (5.3958, 14.8119) (5.3953, 14.8218) (5.3947, 14.8319) (5.3942, 14.8419) (5.3936, 14.852) (5.393, 14.862) (5.3924, 14.8722) (5.3918, 14.8823) (5.3912, 14.8925) (5.3905, 14.9027) (5.3899, 14.9129) (5.3892, 14.9231) (5.3885, 14.9334) (5.3877, 14.9437) (5.387, 14.954) (5.3862, 14.9644) (5.3854, 14.9747) (5.3846, 14.9851) (5.3838, 14.9956) (5.383, 15.006) (5.3821, 15.0165) (5.3813, 15.027) (5.3804, 15.0375) (5.3794, 15.0481) (5.3787, 15.0565) (5.3781, 15.0629) (5.3777, 15.0671) (5.3776, 15.0692) knots 0 0 0 0 0 0 0.00416667 0.00833333 0.0125 0.01666667 0.02083333 0.025 0.02916667 0.03333333 0.0375 0.04166667 0.04583333 0.05 0.05416667 0.05833333 0.0625 0.06666667 0.07083333 0.075 0.07916667 0.08333333 0.0875 0.09166667 0.09583333 0.1 0.10416667 0.10833333 0.1125 0.11666667 0.12083333 0.125 0.12916667 0.13333333 0.1375 0.14166667 0.14583333 0.15 0.15416667 0.15833333 0.1625 0.16666667 0.17083333 0.175 0.17916667 0.18333333 0.1875 0.19166667 0.19583333 0.2 0.20416667 0.20833333 0.2125 0.21666667 0.22083333 0.225 0.22916667 0.23333333 0.2375 0.24166667 0.24583333 0.25 0.25416667 0.25833333 0.2625 0.26666667 0.27083333 0.275 0.27916667 0.28333333 0.2875 0.29166667 0.29583333 0.3 0.30416667 0.30833333 0.3125 0.31666667 0.32083333 0.325 0.32916667 0.33333333 0.3375 0.34166667 0.34583333 0.35 0.35416667 0.35833333 0.3625 0.36666667 0.37083333 0.375 0.37916667 0.38333333 0.3875 0.39166667 0.39583333 0.4 0.40416667 0.40833333 0.4125 0.41666667 0.42083333 0.425 0.42916667 0.43333333 0.4375 0.44166667 0.44583333 0.45 0.45416667 0.45833333 0.4625 0.46666667 0.47083333 0.475 0.47916667 0.48333333 0.4875 0.49166667 0.49583333 0.5 0.50416667 0.50833333 0.5125 0.51666667 0.52083333 0.525 0.52916667 0.53333333 0.5375 0.54166667 0.54583333 0.55 0.55416667 0.55833333 0.5625 0.56666667 0.57083333 0.575 0.57916667 0.58333333 0.5875 0.59166667 0.59583333 0.6 0.60416667 0.60833333 0.6125 0.61666667 0.62083333 0.625 0.62916667 0.63333333 0.6375 0.64166667 0.64583333 0.65 0.65416667 0.65833333 0.6625 0.66666667 0.67083333 0.675 0.67916667 0.68333333 0.6875 0.69166667 0.69583333 0.7 0.70416667 0.70833333 0.7125 0.71666667 0.72083333 0.725 0.72916667 0.73333333 0.7375 0.74166667 0.74583333 0.75 0.75416667 0.75833333 0.7625 0.76666667 0.77083333 0.775 0.77916667 0.78333333 0.7875 0.79166667 0.79583333 0.8 0.80416667 0.80833333 0.8125 0.81666667 0.82083333 0.825 0.82916667 0.83333333 0.8375 0.84166667 0.84583333 0.85 0.85416667 0.85833333 0.8625 0.86666667 0.87083333 0.875 0.87916667 0.88333333 0.8875 0.89166667 0.89583333 0.9 0.90416667 0.90833333 0.9125 0.91666667 0.92083333 0.925 0.92916667 0.93333333 0.9375 0.94166667 0.94583333 0.95 0.95416667 0.95833333 0.9625 0.96666667 0.97083333 0.975 0.97916667 0.98333333 0.9875 0.99166667 0.99583333 1 1 1 1 1 1
  arc A51 (5.3776, 15.0692) -> (4.5069, 15.3521) centre (0, 0) ccw
  spline S43 degree 5 poles (4.5069, 15.3521) (4.5055, 15.3505) (4.5027, 15.3473) (4.4985, 15.3425) (4.493, 15.3361) (4.486, 15.3281) (4.4791, 15.3201) (4.4722, 15.3121) (4.4654, 15.3042) (4.4586, 15.2962) (4.4518, 15.2883) (4.445, 15.2803) (4.4383, 15.2724) (4.4316, 15.2645) (4.4249, 15.2565) (4.4183, 15.2486) (4.4117, 15.2407) (4.4051, 15.2329) (4.3985, 15.225) (4.392, 15.2171) (4.3855, 15.2093) (4.3791, 15.2014) (4.3726, 15.1936) (4.3662, 15.1858) (4.3599, 15.178) (4.3535, 15.1702) (4.3472, 15.1624) (4.3409, 15.1546) (4.3347, 15.1468) (4.3285, 15.1391) (4.3223, 15.1313) (4.3161, 15.1236) (4.31, 15.1159) (4.3039, 15.1082) (4.2978, 15.1005) (4.2918, 15.0928) (4.2858, 15.0851) (4.2798, 15.0775) (4.2738, 15.0698) (4.2679, 15.0622) (4.262, 15.0546) (4.2562, 15.047) (4.2503, 15.0394) (4.2445, 15.0318) (4.2388, 15.0242) (4.233, 15.0167) (4.2273, 15.0092) (4.2216, 15.0016) (4.216, 14.9941) (4.2104, 14.9866) (4.2048, 14.9791) (4.1992, 14.9717) (4.1937, 14.9642) (4.1882, 14.9568) (4.1827, 14.9494) (4.1773, 14.942) (4.1719, 14.9346) (4.1665, 14.9272) (4.1612, 14.9198) (4.1559, 14.9125) (4.1506, 14.9052) (4.1453, 14.8978) (4.1401, 14.8905) (4.1349, 14.8833) (4.1297, 14.876) (4.1246, 14.8687) (4.1195, 14.8615) (4.1144, 14.8543) (4.1094, 14.8471) (4.1044, 14.8399) (4.0994, 14.8328) (4.0944, 14.8256) (4.0895, 14.8185) (4.0846, 14.8114) (4.0798, 14.8043) (4.0749, 14.7972) (4.0701, 14.7901) (4.0654, 14.7831) (4.0606, 14.7761) (4.0559, 14.7691) (4.0512, 14.7621) (4.0466, 14.7551) (4.042, 14.7482) (4.0374, 14.7413) (4.0328, 14.7344) (4.0283, 14.7275) (4.0238, 14.7206) (4.0193, 14.7138) (4.0149, 14.707) (4.0105, 14.7002) (4.0061, 14.6934) (4.0018, 14.6866) (3.9974, 14.6799) (3.9932, 14.6731) (3.9889, 14.6665) (3.9847, 14.6598) (3.9805, 14.6531) (3.9763, 14.6465) (3.9722, 14.6399) (3.9681, 14.6333) (3.964, 14.6267) (3.96, 14.6202) (3.9559, 14.6137) (3.952, 14.6072) (3.948, 14.6007) (3.9441, 14.5942) (3.9402, 14.5878) (3.9363, 14.5814) (3.9325, 14.575) (3.9287, 14.5687) (3.9249, 14.5623) (3.9212, 14.556) (3.9175, 14.5497) (3.9138, 14.5435) (3.9101, 14.5373) (3.9065, 14.5311) (3.9029, 14.5249) (3.8993, 14.5187) (3.8958, 14.5126) (3.8923, 14.5065) (3.8888, 14.5004) (3.8854, 14.4944) (3.882, 14.4883) (3.8786, 14.4824) (3.8752, 14.4764) (3.8719, 14.4704) (3.8686, 14.4645) (3.8654, 14.4587) (3.8621, 14.4528) (3.8589, 14.447) (3.8558, 14.4412) (3.8526, 14.4354) (3.8495, 14.4297) (3.8464, 14.424) (3.8434, 14.4183) (3.8403, 14.4126) (3.8373, 14.407) (3.8344, 14.4014) (3.8314, 14.3959) (3.8285, 14.3903) (3.8257, 14.3848) (3.8228, 14.3794) (3.82, 14.3739) (3.8172, 14.3685) (3.8144, 14.3632) (3.8117, 14.3578) (3.809, 14.3525) (3.8063, 14.3473) (3.8037, 14.342) (3.8011, 14.3368) (3.7985, 14.3316) (3.796, 14.3265) (3.7934, 14.3214) (3.791, 14.3163) (3.7885, 14.3113) (3.7861, 14.3063) (3.7836, 14.3013) (3.7813, 14.2964) (3.7789, 14.2915) (3.7766, 14.2867) (3.7743, 14.2819) (3.7721, 14.2771) (3.7698, 14.2723) (3.7676, 14.2676) (3.7655, 14.263) (3.7633, 14.2583) (3.7612, 14.2537) (3.7591, 14.2492) (3.7571, 14.2447) (3.755, 14.2402) (3.753, 14.2358) (3.7511, 14.2314) (3.7491, 14.227) (3.7472, 14.2227) (3.7453, 14.2185) (3.7435, 14.2142) (3.7416, 14.21) (3.7398, 14.2059) (3.7381, 14.2018) (3.7363, 14.1977) (3.7346, 14.1937) (3.7329, 14.1898) (3.7313, 14.1858) (3.7296, 14.1819) (3.728, 14.1781) (3.7265, 14.1743) (3.7249, 14.1706) (3.7234, 14.1669) (3.7219, 14.1632) (3.7204, 14.1596) (3.719, 14.1561) (3.7176, 14.1525) (3.7162, 14.1491) (3.7149, 14.1457) (3.7136, 14.1423) (3.7123, 14.139) (3.711, 14.1357) (3.7097, 14.1325) (3.7085, 14.1293) (3.7073, 14.1262) (3.7062, 14.1232) (3.7051, 14.1202) (3.704, 14.1172) (3.7029, 14.1143) (3.7018, 14.1114) (3.7008, 14.1086) (3.6998, 14.1059) (3.6988, 14.1032) (3.6979, 14.1006) (3.697, 14.098) (3.6961, 14.0955) (3.6952, 14.093) (3.6944, 14.0906) (3.6936, 14.0883) (3.6928, 14.086) (3.692, 14.0838) (3.6913, 14.0816) (3.6906, 14.0795) (3.6899, 14.0775) (3.6892, 14.0755) (3.6886, 14.0736) (3.688, 14.0717) (3.6874, 14.0699) (3.6869, 14.0682) (3.6863, 14.0665) (3.6858, 14.0649) (3.6853, 14.0634) (3.6849, 14.0619) (3.6845, 14.0606) (3.6841, 14.0592) (3.6837, 14.058) (3.6833, 14.0568) (3.683, 14.0557) (3.6827, 14.0546) (3.6824, 14.0537) (3.6821, 14.0528) (3.6819, 14.0519) (3.6817, 14.0512) (3.6815, 14.0505) (3.6813, 14.0499) (3.6812, 14.0494) (3.6811, 14.0491) (3.681, 14.0488) (3.681, 14.0487) (3.681, 14.0486) knots -1 -1 -1 -1 -1 -1 -0.99583333 -0.99166667 -0.9875 -0.98333333 -0.97916667 -0.975 -0.97083333 -0.96666667 -0.9625 -0.95833333 -0.95416667 -0.95 -0.94583333 -0.94166667 -0.9375 -0.93333333 -0.92916667 -0.925 -0.92083333 -0.91666667 -0.9125 -0.90833333 -0.90416667 -0.9 -0.89583333 -0.89166667 -0.8875 -0.88333333 -0.87916667 -0.875 -0.87083333 -0.86666667 -0.8625 -0.85833333 -0.85416667 -0.85 -0.84583333 -0.84166667 -0.8375 -0.83333333 -0.82916667 -0.825 -0.82083333 -0.81666667 -0.8125 -0.80833333 -0.80416667 -0.8 -0.79583333 -0.79166667 -0.7875 -0.78333333 -0.77916667 -0.775 -0.77083333 -0.76666667 -0.7625 -0.75833333 -0.75416667 -0.75 -0.74583333 -0.74166667 -0.7375 -0.73333333 -0.72916667 -0.725 -0.72083333 -0.71666667 -0.7125 -0.70833333 -0.70416667 -0.7 -0.69583333 -0.69166667 -0.6875 -0.68333333 -0.67916667 -0.675 -0.67083333 -0.66666667 -0.6625 -0.65833333 -0.65416667 -0.65 -0.64583333 -0.64166667 -0.6375 -0.63333333 -0.62916667 -0.625 -0.62083333 -0.61666667 -0.6125 -0.60833333 -0.60416667 -0.6 -0.59583333 -0.59166667 -0.5875 -0.58333333 -0.57916667 -0.575 -0.57083333 -0.56666667 -0.5625 -0.55833333 -0.55416667 -0.55 -0.54583333 -0.54166667 -0.5375 -0.53333333 -0.52916667 -0.525 -0.52083333 -0.51666667 -0.5125 -0.50833333 -0.50416667 -0.5 -0.49583333 -0.49166667 -0.4875 -0.48333333 -0.47916667 -0.475 -0.47083333 -0.46666667 -0.4625 -0.45833333 -0.45416667 -0.45 -0.44583333 -0.44166667 -0.4375 -0.43333333 -0.42916667 -0.425 -0.42083333 -0.41666667 -0.4125 -0.40833333 -0.40416667 -0.4 -0.39583333 -0.39166667 -0.3875 -0.38333333 -0.37916667 -0.375 -0.37083333 -0.36666667 -0.3625 -0.35833333 -0.35416667 -0.35 -0.34583333 -0.34166667 -0.3375 -0.33333333 -0.32916667 -0.325 -0.32083333 -0.31666667 -0.3125 -0.30833333 -0.30416667 -0.3 -0.29583333 -0.29166667 -0.2875 -0.28333333 -0.27916667 -0.275 -0.27083333 -0.26666667 -0.2625 -0.25833333 -0.25416667 -0.25 -0.24583333 -0.24166667 -0.2375 -0.23333333 -0.22916667 -0.225 -0.22083333 -0.21666667 -0.2125 -0.20833333 -0.20416667 -0.2 -0.19583333 -0.19166667 -0.1875 -0.18333333 -0.17916667 -0.175 -0.17083333 -0.16666667 -0.1625 -0.15833333 -0.15416667 -0.15 -0.14583333 -0.14166667 -0.1375 -0.13333333 -0.12916667 -0.125 -0.12083333 -0.11666667 -0.1125 -0.10833333 -0.10416667 -0.1 -0.09583333 -0.09166667 -0.0875 -0.08333333 -0.07916667 -0.075 -0.07083333 -0.06666667 -0.0625 -0.05833333 -0.05416667 -0.05 -0.04583333 -0.04166667 -0.0375 -0.03333333 -0.02916667 -0.025 -0.02083333 -0.01666667 -0.0125 -0.00833333 -0.00416667 0 0 0 0 0 0
  line L86 (3.681, 14.0486) -> (3.6808, 14.048)
  line L87 (3.6808, 14.048) -> (3.4851, 13.301)
  arc A52 (3.4851, 13.301) -> (2.2262, 13.5686) centre (0, 0) ccw
  line L88 (2.2262, 13.5686) -> (2.3513, 14.3306)
  line L89 (2.3513, 14.3306) -> (2.3514, 14.3312)